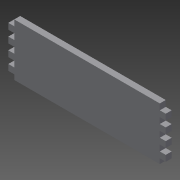
# Autodesk Inventor part: deep_side
Saved by Autodesk Inventor 2014 SP1 (Build 180222100, 222)
## iProperties
Created: 2014-02-21
Part Number: deep_side
Material: Wood (Birch)
Document SubType Name: Modeling
Designer: Chris
Density: 0.55 g/cm^3
Appearance: Birch - Natural Polished
Mass: 853.302 g
Surface Area: 1928.83 cm^2
Volume: 1551.46 cm^3
Author: Chris
Autodesk Inventor part; units mm, degrees
ref_plane "YZ Plane" through (0, 0, 0) normal (1, 0, 0) x (0, 1, 0)
ref_plane "XZ Plane" through (0, 0, 0) normal (0, 1, 0) x (-1, 0, 0)
ref_plane "XY Plane" through (0, 0, 0) normal (0, 0, 1) x (1, 0, 0)
sketch "Sketch1" plane through (0, 0, 0) normal (0, 0, 1) x (1, 0, 0)
  line L0 (0, 0) -> (252.4125, 0)
  line L1 (252.4125, 0) -> (252.4125, 244.475)
  line L2 (252.4125, 244.475) -> (0, 244.475)
  line L3 (0, 244.475) -> (0, 0)
  dimension "d0" = 252.4125
  dimension "d1" = 244.475
  constraints: 8 end point, 2 parallel, 1 horizontal, 1 perpendicular
  measures "d0" distance of L1.end L2.end
  measures "d1" distance of L2.end L0.start
extrude "Extrusion1" add sketch "Sketch1" along normal blind 19.05
sketch "Sketch3" plane through (0, 0, 19.05) normal (0, 0, 1) x (1, 0, 0)
  line L0 (0, 0) -> (252.4125, 0) projected
  line L1 (252.4125, 244.475) -> (0, 244.475) projected
  line L2 (0, 244.475) -> (0, 0) projected
  line L3 (0, 244.475) -> (19.05, 244.475)
  line L4 (19.05, 244.475) -> (19.05, 225.425)
  line L5 (19.05, 225.425) -> (0, 225.425)
  line L6 (0, 225.425) -> (0, 244.475)
  line L7 (19.05, 168.275) -> (0, 168.275)
  line L8 (0, 168.275) -> (0, 149.225)
  line L9 (0, 149.225) -> (19.05, 149.225)
  line L10 (19.05, 149.225) -> (19.05, 168.275)
  line L11 (0, 130.175) -> (19.05, 130.175)
  line L12 (19.05, 130.175) -> (19.05, 111.125)
  line L13 (19.05, 111.125) -> (0, 111.125)
  line L14 (0, 111.125) -> (0, 130.175)
  line L15 (0, 206.375) -> (19.05, 206.375)
  line L16 (19.05, 206.375) -> (19.05, 187.325)
  line L17 (19.05, 187.325) -> (0, 187.325)
  line L18 (0, 187.325) -> (0, 206.375)
  line L19 (0, 92.075) -> (19.05, 92.075)
  line L20 (19.05, 92.075) -> (19.05, 73.025)
  line L21 (19.05, 73.025) -> (0, 73.025)
  line L22 (0, 73.025) -> (0, 92.075)
  line L23 (0, 53.975) -> (19.05, 53.975)
  line L24 (19.05, 53.975) -> (19.05, 34.925)
  line L25 (19.05, 34.925) -> (0, 34.925)
  line L26 (0, 34.925) -> (0, 53.975)
  line L27 (0, 15.875) -> (19.05, 15.875)
  line L28 (19.05, 15.875) -> (19.05, -3.175)
  line L29 (19.05, -3.175) -> (0, -3.175)
  line L30 (0, -3.175) -> (0, 15.875)
  dimension "d4" = 19.05
  dimension "d5" = 19.05
  dimension "d6" = 244.475
  dimension "d7" = 19.05
  dimension "d8" = 19.05
  dimension "d9" = 19.05
  dimension "d10" = 19.05
  dimension "d11" = 19.05
  dimension "d12" = 19.05
  dimension "d13" = 19.05
  dimension "d14" = 19.05
  dimension "d15" = 19.05
  dimension "d16" = 19.05
  dimension "d17" = 19.05
  dimension "d18" = 19.05
  dimension "d19" = 19.05
  dimension "d20" = 19.05
  dimension "d21" = 19.05
  dimension "d22" = 19.05
  dimension "d23" = 19.05
  dimension "d24" = 15.875
  constraints: 56 end point, 14 parallel, 7 horizontal, 7 perpendicular, 6 point on line
  measures "d4" distance of L3.end L4.end
  measures "d5" distance of L4.end L5.end
  measures "d6" distance between parallel lines of L0 L1
  measures "d7" distance between parallel lines of L15 L5
  measures "d8" distance between parallel lines of L17 L15
  measures "d9" distance between parallel lines of L7 L17
  measures "d10" distance between parallel lines of L9 L7
  measures "d11" distance between parallel lines of L11 L9
  measures "d12" distance of L11.end L12.end
  measures "d13" distance of L15.start L15.end
  measures "d14" distance of L7.start L7.end
  measures "d15" distance of L11.start L11.end
  measures "d16" distance between parallel lines of L13 L19
  measures "d17" distance of L19.end L20.end
  measures "d18" distance between parallel lines of L21 L23
  measures "d19" distance of L23.end L24.end
  measures "d20" distance of L27.start L27.end
  measures "d21" distance between parallel lines of L27 L25
  measures "d22" distance of L28.end L29.end
  measures "d23" distance between parallel lines of L27 L29
  measures "d24" distance between parallel lines of L0 L27
extrude "Extrusion2" cut sketch "Sketch3" against normal through all
mirror "Mirror1" about plane through (252.4125, 0, 0) normal (1, 0, 0)
sketch "Sketch6" plane through (0, 0, 19.05) normal (0, 0, 1) x (1, 0, 0)
  line L0 (19.05, 34.925) -> (0, 34.925) projected
  line L1 (0, 34.925) -> (0, 15.875) projected
  line L2 (0, 15.875) -> (19.05, 15.875) projected
  line L3 (19.05, 15.875) -> (19.05, 0) projected
  line L4 (19.05, 0) -> (485.775, 0) projected
  line L5 (485.775, 15.875) -> (485.775, 0) projected
  line L6 (504.825, 15.875) -> (485.775, 15.875) projected
  line L7 (504.825, 34.925) -> (504.825, 15.875) projected
  line L8 (485.775, 34.925) -> (504.825, 34.925) projected
  line L9 (485.775, 53.975) -> (485.775, 34.925) projected
  line L10 (504.825, 53.975) -> (485.775, 53.975) projected
  line L11 (504.825, 73.025) -> (504.825, 53.975) projected
  line L12 (485.775, 73.025) -> (504.825, 73.025) projected
  line L13 (485.775, 92.075) -> (485.775, 73.025) projected
  line L14 (19.05, 92.075) -> (19.05, 73.025) projected
  line L15 (19.05, 73.025) -> (0, 73.025) projected
  line L16 (0, 73.025) -> (0, 53.975) projected
  line L17 (0, 53.975) -> (19.05, 53.975) projected
  line L18 (19.05, 53.975) -> (19.05, 34.925) projected
  line L19 (504.825, 76.2) -> (19.05, 76.2)
  line L20 (19.05, 76.2) -> (485.775, 76.2)
  line L21 (19.05, 244.475) -> (485.775, 244.475) projected
  point P0 (0, 0)
  dimension "d54" = 168.275
  constraints: 4 end point, 2 perpendicular, 2 point on line
  measures "d54" distance between parallel lines of L21 L19
extrude "Extrusion3" cut sketch "Sketch6" against normal through all
body "Solid1"
